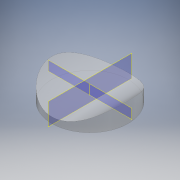
# Autodesk Inventor part: DiscoSuporteInterno
Saved by Autodesk Inventor 2016 (Build 200138000, 138)
## iProperties
Created: 2017-04-03
Part Number: DiscoSuporteInterno
Material: Polycarbonate, Clear
Document SubType Name: Modeling
Designer: Marcelo
Mass: 238.918 g
Surface Area: 326.726 cm^2
Volume: 199.098 cm^3
Density: 1.2 g/cm^3
Appearance: Polycarbonate - Clear
Author: Marcelo
Autodesk Inventor part; units mm, degrees
ref_plane "XZ Plane" through (0, 0, 0) normal (0, 1, 0) x (-1, 0, 0)
ref_plane "XY Plane" through (0, 0, 0) normal (0, 0, 1) x (1, 0, 0)
sketch "Sketch1" plane through (0, 0, 0) normal (0, 0, 1) x (1, 0, 0)
  circle A0 centre (0, 0) radius 65
  dimension "d0" = 130
  constraints: 1 centre point, 1 coincident
  measures "d0" diameter of A0
extrude "Extrusion1" add sketch "Sketch1" along normal blind 25
ref_plane "Work Plane1" through (0, 0, 0) normal (0, 1, 0) x (0, 0, 1)
sketch "Sketch2" plane through (0, 0, 0) normal (0, 1, 0) x (0, 0, 1)
  circle A0 centre (100, 0) radius 100
  line L0 (0, 65) -> (0, -65) projected
  point P0 (0, 0)
  dimension "d4" = 200
  constraints: 1 centre point, 1 tangent
  measures "d4" diameter of A0
extrude "Extrusion2" cut sketch "Sketch2" along normal mid plane 130
sketch "Sketch3" plane through (0, 0, 0) normal (0, 0, -1) x (-1, 0, 0)
  circle A0 centre (0, 0) radius 65
  constraints: 1 centre point, 1 coincident
extrude "Extrusion3" add sketch "Sketch3" along normal blind 10
ref_plane "Work Plane2" through (0, 0, 0) normal (-1, 0, 0) x (0, 0, 1)
body "Solid1"
